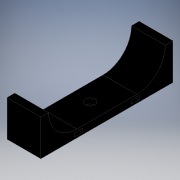
# Autodesk Inventor part: CT_Holder
Saved by Autodesk Inventor 2019 (Build 230136000, 136)
## iProperties
Created: 2021-10-28
Part Number: CT_Holder
Material: Generic
Document SubType Name: Modeling
Designer: Erle
Density: 1 g/cm^3
Appearance: Anodized - Black
Author: Erle
Autodesk Inventor part; units mm, degrees
ref_plane "YZ Plane" through (0, 0, 0) normal (1, 0, 0) x (0, 1, 0)
ref_plane "XZ Plane" through (0, 0, 0) normal (0, 1, 0) x (-1, 0, 0)
ref_plane "XY Plane" through (0, 0, 0) normal (0, 0, 1) x (1, 0, 0)
sketch "Sketch2" plane through (0, 0, 0) normal (1, 0, 0) x (0, 1, 0)
  line L0 (0, 43) -> (0, -43)
  line L1 (0, -43) -> (23.5, -43)
  line L2 (23.5, -43) -> (23.5, -38)
  arc A0 (5, -19.5) -> (23.5, -38) centre (23.5, -19.5) ccw
  line L3 (0, 43) -> (23.5, 43)
  line L4 (23.5, 43) -> (23.5, 38)
  arc A1 (23.5, 38) -> (5, 19.5) centre (23.5, 19.5) ccw
  line L5 (5, 19.5) -> (5, -19.5)
  point P0 (0, 0)
  point P1 (0, 0)
  point P2 (5, 0)
  dimension "d0" = 18.5
  dimension "d1" = 39
  dimension "d2" = 5
  dimension "d3" = 5
  constraints: 12 end point, 4 point on circle, 4 vertical alignment, 3 perpendicular, 2 centre point, 2 midpoint, 2 tangent, 1 coincident, 1 horizontal, 1 horizontal alignment, 1 parallel, 1 vertical
  measures "d0" radius of A1
  measures "d1" distance of L5.start L5.end
  measures "d2" distance of L3.end L4.end
  measures "d3" distance between parallel lines of L0 L5
extrude "Extrusion1" add sketch "Sketch2" along normal blind 22
sketch "Sketch3" plane through (0, 5, 19.5) normal (0, 1, 0) x (1, 0, 0)
  line L0 (0, 39) -> (0, 0) projected
  line L1 (0, -23.5) -> (22, -23.5) projected
  point P0 (0, 19.5)
  point P1 (11, 19.5)
  point P2 (0, 19.5)
  point P3 (11, -23.5)
  constraints: 2 midpoint, 1 horizontal alignment, 1 vertical alignment
hole "Hole1" at (11, 5, 0) direction (0, -1, 0) diameter 3.4 end through all counterbore diameter 6.5 counterbore depth 3.4 clearance for "Socket Head Cap Screw DIN EN ISO 4762" size "M3" standard "DIN"
sketch "Sketch4" plane through (22, 0, 0) normal (1, 0, 0) x (0, 0, -1)
  line L0 (-21, 3.75) -> (-16, 3.75)
  line L1 (-16, 3.75) -> (-16, 1.25)
  line L2 (-16, 1.25) -> (-21, 1.25)
  line L3 (-21, 1.25) -> (-21, 3.75)
  line L4 (16, 3.75) -> (21, 3.75)
  line L5 (21, 3.75) -> (21, 1.25)
  line L6 (21, 1.25) -> (16, 1.25)
  line L7 (16, 1.25) -> (16, 3.75)
  line L8 (-16, 3.75) -> (16, 3.75) construction
  line L9 (-43, 0) -> (43, 0) projected
  line L10 (-3.25, 5) -> (3.25, 5) projected
  line L11 (0, 5) -> (0, 0) construction
  point P0 (0, 0)
  point P1 (0, 3.75)
  point P2 (-16, 2.5)
  point P3 (0, 2.5)
  dimension "d13" = 32
  dimension "d14" = 5
  dimension "d15" = 2.5
  constraints: 20 end point, 5 midpoint, 4 parallel, 2 collinear, 2 horizontal, 2 perpendicular, 2 point on line, 1 horizontal alignment, 1 vertical, 1 vertical alignment
  measures "d13" distance of L0.end L4.start
  measures "d14" distance of L4.start L4.end
  measures "d15" distance of L4.end L5.end
extrude "Extrusion2" cut sketch "Sketch4" against normal through all
body "Solid1"
